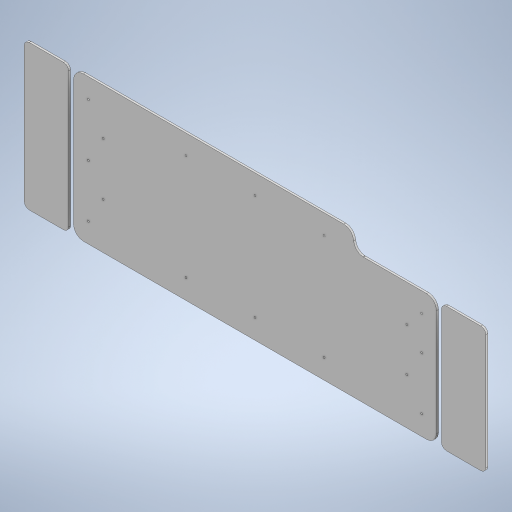
# Autodesk Inventor part: Coffee_Machine_Base
Saved by Autodesk Inventor 2023.5 (Build 275446020, 446B)
## iProperties
Created: 2025-04-17
Part Number: Coffee_Machine_Base
Material: Generic
Document SubType Name: Modeling
Designer: Lucky Sah
Density: 1 g/cm^3
Appearance: Default
Author: Lucky Sah
Autodesk Inventor part; units mm, degrees
ref_plane "YZ Plane" through (0, 0, 0) normal (1, 0, 0) x (0, 1, 0)
ref_plane "XZ Plane" through (0, 0, 0) normal (0, 1, 0) x (-1, 0, 0)
ref_plane "XY Plane" through (0, 0, 0) normal (0, 0, 1) x (1, 0, 0)
sketch "Sketch1" plane through (0, 0, 0) normal (0, 0, 1) x (1, 0, 0)
  line L0 (0, 0) -> (260, 0)
  line L1 (260, 0) -> (260, 128)
  line L2 (220, 147) -> (0, 147)
  line L3 (0, 147) -> (0, 0)
  circle A0 centre (240, 138) radius 8
  arc A1 (229.9934, 137.3628) -> (220, 147) centre (220, 137) ccw
  line L4 (260, 147) -> (260, 147)
  line L5 (240, 128) -> (260, 128)
  line L6 (0, 73.5) -> (260, 73.5)
  line L7 (60, 127) -> (200, 127)
  line L8 (200, 127) -> (200, 20)
  line L9 (200, 20) -> (60, 20)
  line L10 (60, 20) -> (60, 127)
  circle A2 centre (60, 127) radius 1
  circle A3 centre (200, 127) radius 1
  circle A4 centre (200, 20) radius 1
  circle A5 centre (60, 20) radius 1
  circle A6 centre (130, 127) radius 1
  circle A7 centre (130, 20) radius 1
  line L11 (260, 128) -> (264, 128)
  line L12 (264, 128) -> (264, 0)
  line L13 (264, 0) -> (260, 0)
  line L14 (260, 0) -> (260, 128)
  line L15 (0, 147) -> (-4, 147)
  line L16 (-4, 147) -> (-4, 0)
  line L17 (-4, 0) -> (0, 0)
  line L18 (0, 0) -> (0, 147)
  line L19 (-4, 147) -> (-44, 147)
  line L20 (-54, 137) -> (-54, 10)
  line L21 (-44, 0) -> (-4, 0)
  line L22 (-4, 0) -> (-4, 147)
  line L23 (264, 128) -> (304, 128)
  line L24 (314, 118) -> (314, 10)
  line L25 (304, 0) -> (264, 0)
  line L26 (264, 0) -> (264, 128)
  arc A8 (-44, 147) -> (-54, 137) centre (-44, 137) ccw
  arc A9 (-54, 10) -> (-44, 0) centre (-44, 10) ccw
  arc A10 (304, 0) -> (314, 10) centre (304, 10) ccw
  arc A11 (314, 118) -> (304, 128) centre (304, 118) ccw
  arc A12 (239.4838, 127.9864) -> (240, 128) centre (239.4816, 137.9024) ccw
  line L27 (299, 128) -> (299, 0)
  line L28 (284, 128) -> (284, 0)
  line L29 (-39, 147) -> (-39, 0)
  line L30 (-24, 147) -> (-24, 0)
  arc A13 (229.9934, 137.3628) -> (239.4838, 127.9864) centre (240, 138) ccw
  circle A14 centre (-39, 73.5) radius 1
  circle A15 centre (-39, 20) radius 1
  circle A16 centre (-39, 127) radius 1
  circle A17 centre (299, 108) radius 1
  circle A18 centre (299, 20) radius 1
  circle A19 centre (299, 73.5) radius 1
  circle A20 centre (284, 90.75) radius 1
  circle A21 centre (284, 46.75) radius 1
  circle A22 centre (-24, 100.25) radius 1
  circle A23 centre (-24, 46.75) radius 1
  line L31 (-64, 147) -> (-99, 147)
  line L32 (-104, 142) -> (-104, 5)
  line L33 (-99, 0) -> (-64, 0)
  line L34 (-59, 5) -> (-59, 142)
  line L35 (324, 127) -> (359, 127)
  line L36 (364, 122) -> (364, 5)
  line L37 (359, 0) -> (324, 0)
  line L38 (319, 5) -> (319, 122)
  arc A24 (364, 122) -> (359, 127) centre (359, 122) ccw
  arc A25 (324, 127) -> (319, 122) centre (324, 122) ccw
  arc A26 (319, 5) -> (324, 0) centre (324, 5) ccw
  arc A27 (359, 0) -> (364, 5) centre (359, 5) ccw
  arc A28 (-64, 0) -> (-59, 5) centre (-64, 5) ccw
  arc A29 (-104, 5) -> (-99, 0) centre (-99, 5) ccw
  arc A30 (-99, 147) -> (-104, 142) centre (-99, 142) ccw
  arc A31 (-59, 142) -> (-64, 147) centre (-64, 142) ccw
  point P0 (230, 135)
  point P1 (260, 67.5)
  point P2 (-54, 0)
  point P3 (314, 0)
  point P4 (-4, 0)
  point P5 (264, 0)
  point P6 (-4, 0)
  point P7 (264, 0)
  point P8 (-104, 0)
  point P9 (-59, 0)
  point P10 (364, 0)
  point P11 (319, 0)
  dimension "d2" = 16
  dimension "d3" = 20
  dimension "d4" = 138
  dimension "d6" = 260
  dimension "d7" = 147
  dimension "d8" = 10
  dimension "d11" = 19
  dimension "d16" = 20
  dimension "d17" = 20
  dimension "d18" = 60
  dimension "d19" = 60
  dimension "d20" = 2
  dimension "d21" = 2
  dimension "d22" = 2
  dimension "d23" = 2
  dimension "d24" = 140
  dimension "d25" = 107
  dimension "d26" = 2
  dimension "d27" = 2
  dimension "d29" = 70
  dimension "d30" = 4
  dimension "d31" = 4
  dimension "d32" = 50
  dimension "d33" = 50
  dimension "d34" = 10
  dimension "d35" = 368
  dimension "d37" = 15
  dimension "d38" = 15
  dimension "d39" = 15
  dimension "d40" = 15
  dimension "d41" = 2
  dimension "d42" = 73.5
  dimension "d43" = 2
  dimension "d44" = 2
  dimension "d45" = 2
  dimension "d46" = 2
  dimension "d47" = 20
  dimension "d48" = 20
  dimension "d49" = 2
  dimension "d50" = 2
  dimension "d51" = 2
  dimension "d52" = 2
  dimension "d53" = 53.5
  dimension "d54" = 26.75
  dimension "d55" = 26.75
  dimension "d56" = 17.25
  dimension "d57" = 26.75
  dimension "d58" = 20
  dimension "d59" = 45
  dimension "d60" = 45
  dimension "d61" = 34.5
  dimension "d62" = 5
  dimension "d63" = 5
  dimension "d66" = 5
  dimension "d67" = 5
  constraints: 80 end point, 32 centre point, 31 point on circle, 31 point on line, 25 tangent, 16 parallel, 14 perpendicular, 9 equal radius, 8 horizontal, 8 midpoint, 4 coincident, 1 collinear
  measures "d2" diameter of A0
  measures "d3" distance from line of L1 A0.centre
  measures "d4" distance from line of L0 A0.centre
  measures "d6" distance from line of point (260, 67.5) L3
  measures "d7" distance between parallel lines of L0 L2
  measures "d8" radius of A1
  measures "d11" distance between parallel lines of L2 L5
  measures "d16" distance between parallel lines of L7 L2
  measures "d17" distance between parallel lines of L0 L9
  measures "d18" distance between parallel lines of L3 L10
  measures "d19" distance between parallel lines of L1 L8
  measures "d20" diameter of A2
  measures "d21" diameter of A3
  measures "d22" diameter of A4
  measures "d23" diameter of A5
  measures "d24" distance between parallel lines of L8 L10
  measures "d25" distance between parallel lines of L9 L7
  measures "d26" diameter of A6
  measures "d27" diameter of A7
  measures "d29" distance from line of L8 A7.centre
  measures "d30" distance between parallel lines of L12 L1
  measures "d31" distance between parallel lines of L16 L3
  measures "d32" distance between parallel lines of L20 L16
  measures "d33" distance between parallel lines of L24 L12
  measures "d34" radius of A8
  measures "d35" distance between parallel lines of L24 L20
  measures "d37" distance between parallel lines of L29 L20
  measures "d38" distance between parallel lines of L29 L30
  measures "d39" distance between parallel lines of L27 L24
  measures "d40" distance between parallel lines of L27 L28
  measures "d41" diameter of A14
  measures "d42" distance between parallel lines of L0 L6
  measures "d43" diameter of A15
  measures "d44" diameter of A17
  measures "d45" diameter of A18
  measures "d46" diameter of A19
  measures "d47" distance from line of A17.centre L23
  measures "d48" distance from line of L25 A18.centre
  measures "d49" diameter of A20
  measures "d50" diameter of A21
  measures "d51" diameter of A22
  measures "d52" diameter of A23
  measures "d53" distance between parallel lines of L6 L7
  measures "d54" distance from line of L6 A22.centre
  measures "d55" distance from line of A23.centre L9
  measures "d56" distance from line of L6 A20.centre
  measures "d57" distance from line of L6 A21.centre
  measures "d58" distance between parallel lines of L30 L16
  measures "d59" distance of point (-59, 0) point (-104, 0)
  measures "d60" distance of point (364, 0) point (319, 0)
  measures "d61" distance from line of L6 A17.centre
  measures "d62" radius of A24
  measures "d63" radius of A25
  measures "d66" distance between parallel lines of L34 L20
  measures "d67" distance between parallel lines of L38 L24
extrude "Extrusion1" add sketch "Sketch1" along normal blind 2 contours L3 L6 L10 A5 L9 A7 A4 L8 L1 L0 | L17 L16 L15 L3 | L1 L11 L12 L13 | L3 L2 A1 A13 A12 L5 L1 L6 L8 A3 L7 A6 A2 L10 | L21 L30 A23 A22 L19 L16 | L12 L23 L28 A20 A21 L25 | L10 A2 L7 A6 A3 L8 L6 | L6 L8 A4 L9 A7 A5 L10 | L21 L29 A15 A14 A16 L19 L30 A22 A23 | L28 A21 A20 L23 L27 A17 A19 A18 L25 | L21 A9 L20 A8 L19 L29 A16 A14 A15 | L27 A18 A19 A17 L23 A11 L24 A10 L25
extrude "Extrusion2" add sketch "Sketch1" along normal blind 2 contours A31 L34 A28 L33 A29 L32 A30 L31 | L35 A24 L36 A27 L37 A26 L38 A25
body "Solid1"
